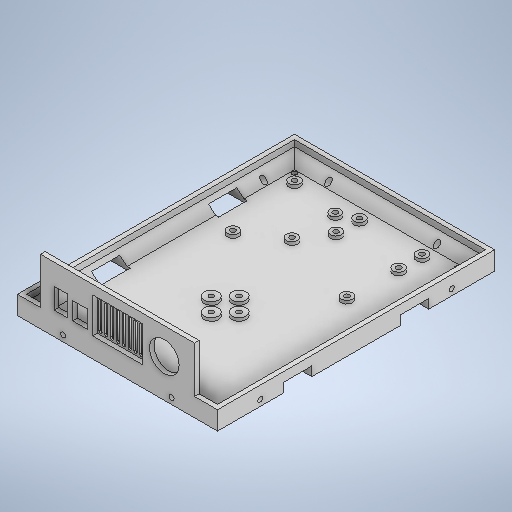
# Autodesk Inventor part: base_v2
Saved by Autodesk Inventor 2025.1 (Build 291241000, 241)
## iProperties
Created: 2024-08-06
Part Number: base_v2
Material: Genérico
Document SubType Name: Modeling
Designer: andre
Density: 1 g/cm^3
Appearance: Valor por defecto
Author: andre
Autodesk Inventor part; units mm, degrees
ref_plane "YZ Plane" through (0, 0, 0) normal (1, 0, 0) x (0, 1, 0)
ref_plane "XZ Plane" through (0, 0, 0) normal (0, 1, 0) x (-1, 0, 0)
ref_plane "XY Plane" through (0, 0, 0) normal (0, 0, 1) x (1, 0, 0)
sketch "base" plane through (0, 0, 0) normal (0, 1, 0) x (-1, 0, 0)
  line L0 (0, 0) -> (130, 0)
  line L1 (130, 0) -> (130, -180)
  line L2 (130, -180) -> (0, -180)
  line L3 (0, -180) -> (0, 0)
  dimension "d53" = 130
  dimension "d54" = 180
  constraints: 8 end point, 2 parallel, 1 horizontal, 1 perpendicular
  measures "d53" distance of L1.end L2.end
  measures "d54" distance of L0.end L1.end
extrude "Extrusión6" add sketch "base" along normal blind 2
sketch "Boceto10" plane through (0, 2, 0) normal (0, 1, 0) x (1, 0, 0)
  line L0 (-130, 180) -> (-130, 0) projected
  line L1 (0, 180) -> (-130, 180) projected
  line L2 (-130, 0) -> (0, 0)
  line L3 (0, 0) -> (0, 180)
  line L4 (0, 180) -> (-130, 180)
  line L5 (-130, 180) -> (-130, 0)
  line L6 (-3, 3) -> (-127, 3)
  line L7 (-127, 3) -> (-127, 177)
  line L8 (-127, 177) -> (-3, 177)
  line L9 (-3, 177) -> (-3, 3)
  dimension "d57" = 3
  constraints: 16 end point, 4 parallel, 2 perpendicular, 1 horizontal, 3 other
  measures "d57" distance between parallel lines of L2 L6
extrude "Extrusión7" add sketch "Boceto10" along normal blind 10
sketch "Boceto17" plane through (0, 12, 0) normal (0, 1, 0) x (1, 0, 0)
  line L0 (-3, 177) -> (-3, 3) projected
  line L1 (0, 0) -> (0, 180) construction
  line L2 (-3, 3) -> (-127, 3) construction
  line L3 (0, 0) -> (-15, 0) construction
  line L4 (-15, 0) -> (-15, 3) construction
  line L5 (-15, 3) -> (0, 3) construction
  line L6 (0, 3) -> (0, 0) construction
  line L7 (-130, 180) -> (-130, 0) construction
  line L8 (-130, 0) -> (-115, 0) construction
  line L9 (-115, 0) -> (-115, 3) construction
  line L10 (-115, 3) -> (-130, 3) construction
  line L11 (-130, 3) -> (-130, 0) construction
  line L12 (-15, 0) -> (-115, 0)
  line L13 (-115, 0) -> (-115, 3)
  line L14 (-115, 3) -> (-15, 3)
  line L15 (-15, 3) -> (-15, 0)
  dimension "d176" = 15
  dimension "d177" = 15
  constraints: 24 end point, 6 parallel, 3 horizontal, 3 perpendicular, 2 point on line
  measures "d176" distance of L4.end L5.end
  measures "d177" distance of L10.end L9.end
extrude "Extrusión13" add sketch "Boceto17" along normal blind 30
sketch "Boceto16" plane through (0, 2, 0) normal (0, 1, 0) x (1, 0, 0)
  line L0 (-3, 177) -> (-127, 177) projected
  line L1 (-3, 3) -> (-3, 177) projected
  line L2 (-127, 177) -> (-3, 177)
  line L3 (-3, 177) -> (-3, 3)
  line L4 (-3, 3) -> (-127, 3)
  line L5 (-127, 3) -> (-127, 177)
  line L6 (-120, 170) -> (-10, 170)
  line L7 (-10, 170) -> (-10, 10)
  line L8 (-10, 10) -> (-120, 10)
  line L9 (-120, 10) -> (-120, 170)
  point P0 (0, 0)
  dimension "d170" = 7
  constraints: 16 end point, 4 parallel, 2 perpendicular, 1 horizontal, 3 other
  measures "d170" distance between parallel lines of L5 L9
extrude "Extrusión12" add sketch "Boceto16" along normal blind 6
sketch "Boceto15" plane through (0, 0, 0) normal (0, -1, 0) x (1, 0, 0)
  line L0 (-130, 0) -> (0, 0) projected
  line L1 (-130, -180) -> (-130, 0) projected
  line L2 (0, 0) -> (-130, 0)
  line L3 (-130, 0) -> (-130, -180)
  line L4 (-130, -180) -> (0, -180)
  line L5 (0, -180) -> (0, 0)
  line L6 (0, -180) -> (-1.1, -180) construction
  line L7 (0, -157.5704) -> (0, -180) construction
  line L8 (0, -180) -> (-12, -180) construction
  line L9 (-12, -180) -> (-12, -168) construction
  line L10 (-12, -168) -> (0, -168) construction
  line L11 (0, -168) -> (0, -180) construction
  line L12 (0, 0) -> (-12, 0) construction
  line L13 (-12, 0) -> (-12, -12) construction
  line L14 (-12, -12) -> (0, -12) construction
  line L15 (0, -12) -> (0, 0) construction
  line L16 (-130, 0) -> (-118, 0) construction
  line L17 (-118, 0) -> (-118, -12) construction
  line L18 (-118, -12) -> (-130, -12) construction
  line L19 (-130, -12) -> (-130, 0) construction
  line L20 (-130, -180) -> (-118, -180) construction
  line L21 (-118, -180) -> (-118, -168) construction
  line L22 (-118, -168) -> (-130, -168) construction
  line L23 (-130, -168) -> (-130, -180) construction
  circle A0 centre (-12, -168) radius 1.625
  circle A1 centre (-118, -168) radius 1.625
  circle A2 centre (-12, -12) radius 1.625
  circle A3 centre (-118, -12) radius 1.625
  dimension "d155" = 12
  dimension "d156" = 12
  dimension "d157" = 12
  dimension "d158" = 12
  dimension "d159" = 12
  dimension "d160" = 12
  dimension "d161" = 12
  dimension "d162" = 12
  dimension "d163" = 3.25
  dimension "d164" = 3.25
  dimension "d165" = 3.25
  dimension "d166" = 3.25
  constraints: 44 end point, 10 parallel, 6 horizontal, 5 perpendicular, 4 centre point, 4 coincident
  measures "d155" distance of L9.end L10.end
  measures "d156" distance of L8.end L9.end
  measures "d157" distance of L14.end L13.end
  measures "d158" distance of L13.end L12.end
  measures "d159" distance of L17.end L18.end
  measures "d160" distance of L16.end L17.end
  measures "d161" distance of L22.end L21.end
  measures "d162" distance of L21.end L20.end
  measures "d163" diameter of A0
  measures "d164" diameter of A1
  measures "d165" diameter of A2
  measures "d166" diameter of A3
extrude "Extrusión11" cut sketch "Boceto15" against normal blind 30 contours A0 | A1 | A2 | A3
sketch "Boceto11" plane through (0, 2, 0) normal (0, 1, 0) x (1, 0, 0)
  line L0 (-127, 3) -> (-127, 177) projected
  line L1 (-3, 177) -> (-3, 3) projected
  line L2 (-127, 3) -> (-3, 3)
  line L3 (-3, 3) -> (-3, 177)
  line L4 (-3, 177) -> (-127, 177)
  line L5 (-127, 177) -> (-127, 3)
  line L6 (-130, 0) -> (0, 0) projected
  line L7 (-130, 0) -> (0, 0)
  line L8 (0, 0) -> (0, 180.7986)
  line L9 (0, 180.7986) -> (-130, 180.7986)
  line L10 (-130, 180.7986) -> (-130, 0)
  line L11 (-9, 9) -> (-121, 9) construction
  line L12 (-121, 9) -> (-121, 171) construction
  line L13 (-121, 171) -> (-9, 171) construction
  line L14 (-9, 171) -> (-9, 9) construction
  line L15 (-121, 171) -> (-9, 171) construction
  line L16 (-9, 171) -> (-9, 108) construction
  line L17 (-9, 108) -> (-121, 108) construction
  line L18 (-121, 108) -> (-121, 171) construction
  line L19 (-118, 111) -> (-16, 111) construction
  line L20 (-16, 111) -> (-16, 165) construction
  line L21 (-16, 165) -> (-118, 165) construction
  line L22 (-118, 165) -> (-118, 111) construction
  line L23 (-121, 108) -> (-117.6431, 108) construction
  line L24 (-16, 165) -> (-30, 165) construction
  line L25 (-30, 165) -> (-30, 162) construction
  line L26 (-30, 162) -> (-16, 162) construction
  line L27 (-16, 162) -> (-16, 165) construction
  line L28 (-30, 162) -> (-30, 114) construction
  line L29 (-30, 162) -> (18, 162) construction
  line L30 (-30, 162) -> (-112, 162) construction
  line L31 (-30, 162) -> (52, 162) construction
  line L32 (-30, 114) -> (-104, 114) construction
  line L33 (-30, 114) -> (44, 114) construction
  circle A0 centre (-104, 114) radius 1.625 construction
  circle A1 centre (-112, 162) radius 1.625 construction
  circle A2 centre (-30, 114) radius 1.625 construction
  line L34 (-30, 114) -> (-80.8, 114) construction
  line L35 (-80.8, 114) -> (-80.8, 129.2) construction
  line L36 (-80.8, 129.2) -> (-30, 129.2) construction
  line L37 (-30, 129.2) -> (-30, 114) construction
  circle A3 centre (-80.8, 129.2) radius 1.625 construction
  line L38 (-30, 162) -> (-80.8, 162) construction
  line L39 (-80.8, 162) -> (-80.8, 157.3) construction
  line L40 (-80.8, 157.3) -> (-30, 157.3) construction
  line L41 (-30, 157.3) -> (-30, 162) construction
  circle A4 centre (-80.8, 157.3) radius 1.5 construction
  line L42 (-30, 162) -> (-29.1, 162) construction
  circle A5 centre (-29.1, 162) radius 1.625 construction
  line L43 (-65, 9) -> (-65, 70) construction
  line L44 (-65, 9) -> (-4, 9) construction
  line L45 (-29.1, 162) -> (-69.74, 162) construction
  line L46 (-69.74, 162) -> (-69.74, 146.76) construction
  line L47 (-69.74, 146.76) -> (-29.1, 146.76) construction
  line L48 (-29.1, 146.76) -> (-29.1, 162) construction
  circle A6 centre (-69.74, 146.76) radius 1.625 construction
  circle A7 centre (-69.74, 162) radius 1.625 construction
  circle A8 centre (-29.1, 146.76) radius 1.625 construction
  circle A9 centre (-65, 70) radius 9 construction
  circle A10 centre (-65, 70) radius 51 construction
  circle A11 centre (-65, 70) radius 45 construction
  circle A12 centre (-65, 61) radius 1.625 construction
  line L49 (-65, 61) -> (-65, 79) construction
  circle A13 centre (-65, 79) radius 1.625 construction
  circle A14 centre (-56, 70) radius 1.625 construction
  circle A15 centre (-74, 70) radius 1.625 construction
  circle A16 centre (-65, 61) radius 4.625
  circle A17 centre (-74, 70) radius 4.625
  circle A18 centre (-65, 79) radius 4.625
  circle A19 centre (-56, 70) radius 4.625
  circle A20 centre (-30, 114) radius 3.625
  circle A21 centre (-29.1, 146.76) radius 3.625
  circle A22 centre (-104, 114) radius 3.625
  circle A23 centre (-80.8, 129.2) radius 3.625
  circle A24 centre (-112, 162) radius 3.625
  circle A25 centre (-80.8, 157.3) radius 3.5
  circle A26 centre (-69.74, 146.76) radius 3.625
  circle A27 centre (-69.74, 162) radius 3.625
  circle A28 centre (-29.1, 162) radius 3.625
  point P0 (-118, 111)
  point P1 (-27.9651, 111)
  point P2 (-32.0349, 111)
  point P3 (-31.1349, 165)
  point P4 (-27.0651, 165)
  point P5 (-71.7749, 165)
  point P6 (-67.7051, 165)
  point P7 (-114.0349, 165)
  point P8 (-109.9651, 165)
  dimension "d60" = 6
  dimension "d64" = 102
  dimension "d65" = 54
  dimension "d71" = 3
  dimension "d73" = 3
  dimension "d74" = 14
  dimension "d75" = 3
  dimension "d76" = 48
  dimension "d78" = 82
  dimension "d80" = 74
  dimension "d86" = 50.8
  dimension "d87" = 15.2
  dimension "d88" = 3.25
  dimension "d89" = 50.8
  dimension "d90" = 4.7
  dimension "d91" = 3
  dimension "d92" = 0.9
  dimension "d96" = 61
  dimension "d97" = 40.64
  dimension "d98" = 15.24
  dimension "d99" = 3.25
  dimension "d100" = 3.25
  dimension "d101" = 3.25
  dimension "d102" = 18
  dimension "d103" = 102
  dimension "d104" = 6
  dimension "d105" = 3.25
  dimension "d106" = 3.25
  dimension "d107" = 3.25
  dimension "d108" = 3.25
  dimension "d109" = 3
  dimension "d110" = 3
  dimension "d111" = 3
  dimension "d112" = 3
  dimension "d113" = 2
  dimension "d114" = 2
  dimension "d115" = 2
  dimension "d116" = 2
  dimension "d117" = 2
  dimension "d118" = 2
  dimension "d119" = 2
  dimension "d120" = 2
  dimension "d121" = 2
  dimension "d380" = 3.25
  dimension "d381" = 3.25
  dimension "d382" = 3.25
  dimension "d383" = 3.25
  constraints: 94 end point, 29 centre point, 23 coincident, 18 parallel, 15 horizontal, 10 perpendicular, 4 equal length, 4 point on circle, 3 point on line, 1 midpoint, 1 vertical, 3 other
  measures "d60" distance between parallel lines of L2 L11
  measures "d64" distance of L21.end L20.end
  measures "d65" distance of L20.end L19.end
  measures "d71" distance from line of L18 point (-118, 111)
  measures "d73" distance from line of L23 point (-118, 111)
  measures "d74" distance of L26.end L25.end
  measures "d75" distance of L25.end L24.end
  measures "d76" distance of L28.start L28.end
  measures "d78" distance of L28.start L30.end
  measures "d80" distance of L32.start L32.end
  measures "d86" distance of L35.end L36.end
  measures "d87" distance of L34.end L35.end
  measures "d88" diameter of A3
  measures "d89" distance of L40.end L39.end
  measures "d90" distance of L39.end L38.end
  measures "d91" diameter of A4
  measures "d92" distance of L38.start L42.end
  measures "d96" distance of point (-65, 70) L43.start
  measures "d97" distance of L47.end L46.end
  measures "d98" distance of L46.end L45.end
  measures "d99" diameter of A6
  measures "d100" diameter of A7
  measures "d101" diameter of A8
  measures "d102" diameter of A9
  measures "d103" diameter of A10
  measures "d104" radial gap between concentric circles of A10 A11
  measures "d105" diameter of A12
  measures "d106" diameter of A13
  measures "d107" diameter of A14
  measures "d108" diameter of A15
  measures "d109" radial gap between concentric circles of A12 A16
  measures "d110" radial gap between concentric circles of A15 A17
  measures "d111" radial gap between concentric circles of A13 A18
  measures "d112" radial gap between concentric circles of A14 A19
  measures "d113" radial gap between concentric circles of A2 A20
  measures "d114" radial gap between concentric circles of A8 A21
  measures "d115" radial gap between concentric circles of A0 A22
  measures "d116" radial gap between concentric circles of A3 A23
  measures "d117" radial gap between concentric circles of A1 A24
  measures "d118" radial gap between concentric circles of A4 A25
  measures "d119" radial gap between concentric circles of A6 A26
  measures "d120" radial gap between concentric circles of A7 A27
  measures "d121" radial gap between concentric circles of A5 A28
  measures "d380" diameter of A5
  measures "d381" diameter of A1
  measures "d382" diameter of A0
  measures "d383" diameter of A2
extrude "Extrusión8" add sketch "Boceto11" along normal blind 2 contours A16 | A17 | A18 | A19 | A20 | A21 | A22 | A23 | A24 | A25 | A26 | A27 | A28
chamfer "Chaflán1" distance 7 distance2 6 4 edges at (-120, 8, -90) (-65, 8, -170) (-10, 8, -90) (-65, 8, -10) measured on face at (-124.6667, 8, -116.6667)
sketch "Boceto20" plane through (-130, 0, -180) normal (-1, 0, 0) x (0, 0, 1)
  line L0 (180, 0) -> (0, 0) projected
  line L1 (177, 12) -> (3, 12) projected
  line L2 (3, 8) -> (177, 8) projected
  line L3 (3, 8) -> (177, 8)
  line L4 (90, 8) -> (90, 0) construction
  line L5 (180, 0) -> (180, 12) construction
  circle A0 centre (27.8, 4) radius 1.625
  circle A1 centre (152.2, 4) radius 1.625
  line L6 (180, 0) -> (152.2, 0) construction
  line L7 (152.2, 0) -> (152.2, 4) construction
  line L8 (152.2, 4) -> (180, 4) construction
  line L9 (180, 4) -> (180, 0) construction
  point P0 (90, 4)
  point P1 (90, 12)
  dimension "d237" = 3.25
  dimension "d238" = 3.25
  dimension "d307" = 62.2
  dimension "d308" = 62.2
  dimension "d405" = 4
  dimension "d406" = 4
  constraints: 12 end point, 4 midpoint, 2 centre point, 2 horizontal, 2 parallel, 2 perpendicular
  measures "d237" diameter of A0
  measures "d238" diameter of A1
  measures "d307" distance of point (90, 4) A0.centre
  measures "d308" distance from line of L7.end L4
  measures "d405" distance from line of L0 L7.end
  measures "d406" distance from line of L0 A0.centre
extrude "Extrusión16" cut sketch "Boceto20" against normal blind 140
sketch "Boceto18" plane through (-130, 0, 0) normal (0, 0, 1) x (1, 0, 0)
  line L0 (0, 42) -> (0, 0) construction
  line L1 (0, 0) -> (35, 0) construction
  line L2 (36, 15) -> (45.4, 15)
  line L3 (45.4, 15) -> (45.4, 26.4)
  line L4 (45.4, 26.4) -> (36, 26.4)
  line L5 (36, 26.4) -> (36, 15)
  line L6 (130, 0) -> (95.45, 0) construction
  line L7 (95.45, 0) -> (95.45, 24.65) construction
  line L8 (95.45, 24.65) -> (130, 24.65) construction
  line L9 (130, 24.65) -> (130, 0) construction
  circle A0 centre (95.45, 24.65) radius 9.65
  line L10 (0, 0) -> (130, 0) construction
  line L11 (130, 0) -> (130, 60) construction
  line L12 (130, 60) -> (0, 60) construction
  line L13 (0, 60) -> (0, 0) construction
  line L14 (23, 0) -> (1, 0) construction
  line L15 (24, 15) -> (32.4, 15)
  line L16 (32.4, 15) -> (32.4, 28.4)
  line L17 (32.4, 28.4) -> (24, 28.4)
  line L18 (24, 28.4) -> (24, 15)
  line L19 (20, 37) -> (110, 37)
  line L20 (110, 12) -> (20, 12)
  line L21 (20, 37) -> (20, 12)
  line L22 (110, 37) -> (110, 12)
  line L23 (42.5275, 15) -> (41.0275, 15)
  line L24 (20, 15) -> (110, 15) construction
  line L25 (85.8, 24.65) -> (85.8, 15) construction
  line L26 (50, 15) -> (79.4, 15) construction
  line L27 (50.9, 33.1) -> (50.9, 16)
  line L28 (52.9, 16) -> (52.9, 33.1)
  arc A1 (50.9, 16) -> (52.9, 16) centre (51.9, 16) ccw
  arc A2 (52.9, 33.1) -> (50.9, 33.1) centre (51.9, 33.1) ccw
  line L29 (54.7, 33.1) -> (54.7, 16)
  line L30 (56.7, 16) -> (56.7, 33.1)
  arc A3 (54.7, 16) -> (56.7, 16) centre (55.7, 16) ccw
  line L31 (58.5, 33.1) -> (58.5, 16)
  line L32 (60.5, 16) -> (60.5, 33.1)
  arc A4 (58.5, 16) -> (60.5, 16) centre (59.5, 16) ccw
  arc A5 (60.5, 33.1) -> (58.5, 33.1) centre (59.5, 33.1) ccw
  arc A6 (62.3, 16) -> (64.3, 16) centre (63.3, 16) ccw
  line L33 (64.3, 16) -> (64.3, 33.1)
  line L34 (62.3, 33.1) -> (62.3, 16)
  line L35 (66.1, 33.1) -> (66.1, 16)
  line L36 (68.1, 16) -> (68.1, 33.1)
  arc A7 (66.1, 16) -> (68.1, 16) centre (67.1, 16) ccw
  arc A8 (68.1, 33.1) -> (66.1, 33.1) centre (67.1, 33.1) ccw
  arc A9 (69.9, 16) -> (71.9, 16) centre (70.9, 16) ccw
  line L37 (71.9, 16) -> (71.9, 33.1)
  line L38 (69.9, 33.1) -> (69.9, 16)
  line L39 (73.7, 33.1) -> (73.7, 16)
  line L40 (75.7, 16) -> (75.7, 33.1)
  arc A10 (73.7, 16) -> (75.7, 16) centre (74.7, 16) ccw
  arc A11 (75.7, 33.1) -> (73.7, 33.1) centre (74.7, 33.1) ccw
  arc A12 (77.5, 16) -> (79.5, 16) centre (78.5, 16) ccw
  line L41 (79.5, 16) -> (79.5, 33.1)
  line L42 (77.5, 33.1) -> (77.5, 16)
  arc A13 (56.7, 33.1) -> (54.7, 33.1) centre (55.7, 33.1) ccw
  arc A14 (64.3, 33.1) -> (62.3, 33.1) centre (63.3, 33.1) ccw
  arc A15 (71.9, 33.1) -> (69.9, 33.1) centre (70.9, 33.1) ccw
  arc A16 (79.5, 33.1) -> (77.5, 33.1) centre (78.5, 33.1) ccw
  point P0 (95.45, 15)
  point P1 (105.1, 24.65)
  point P2 (95.45, 15)
  dimension "d182" = 9.4
  dimension "d186" = 34.55
  dimension "d188" = 19.3
  dimension "d189" = 60
  dimension "d190" = 15
  dimension "d191" = 8.4
  dimension "d192" = 13.4
  dimension "d193" = 23
  dimension "d195" = 12
  dimension "d196" = 20
  dimension "d198" = 20
  dimension "d201" = 15
  dimension "d202" = 24
  dimension "d203" = 15
  dimension "d204" = 36
  dimension "d205" = 1.5
  dimension "d207" = 50
  dimension "d250" = 25
  dimension "d407" = 11.4
  dimension "d408" = 2
  dimension "d409" = 2
  dimension "d410" = 2
  dimension "d411" = 2
  dimension "d412" = 2
  dimension "d413" = 2
  dimension "d414" = 2
  dimension "d415" = 2
  dimension "d424" = 5.5
  dimension "d425" = 1.8
  dimension "d426" = 1.8
  dimension "d427" = 1.8
  dimension "d428" = 1.8
  dimension "d429" = 1.8
  dimension "d430" = 1.8
  dimension "d431" = 1.8
  constraints: 90 end point, 35 point on circle, 25 tangent, 17 centre point, 17 parallel, 7 perpendicular, 7 point on line, 6 horizontal, 3 coincident, 1 vertical
  measures "d182" distance of L4.end L3.end
  measures "d186" distance of L7.end L8.end
  measures "d188" diameter of A0
  measures "d189" distance of L11.end L10.end
  measures "d190" distance of L6.end point (95.45, 15)
  measures "d191" distance of L17.end L16.end
  measures "d192" distance of L16.end L15.end
  measures "d193" distance between parallel lines of L12 L19
  measures "d195" distance between parallel lines of L10 L20
  measures "d196" distance between parallel lines of L21 L0
  measures "d198" distance between parallel lines of L9 L22
  measures "d201" distance between parallel lines of L1 L15
  measures "d202" distance between parallel lines of L0 L18
  measures "d203" distance between parallel lines of L10 L2
  measures "d204" distance between parallel lines of L0 L5
  measures "d205" distance of L23.start L23.end
  measures "d207" distance from line of L0 L26.start
  measures "d250" distance between parallel lines of L20 L19
  measures "d407" distance between parallel lines of L4 L2
  measures "d408" distance between parallel lines of L28 L27
  measures "d409" distance between parallel lines of L30 L29
  measures "d410" distance between parallel lines of L32 L31
  measures "d411" distance between parallel lines of L33 L34
  measures "d412" distance between parallel lines of L36 L35
  measures "d413" distance between parallel lines of L37 L38
  measures "d414" distance between parallel lines of L40 L39
  measures "d415" distance between parallel lines of L41 L42
  measures "d424" distance between parallel lines of L3 L27
  measures "d425" distance between parallel lines of L29 L28
  measures "d426" distance between parallel lines of L30 L31
  measures "d427" distance between parallel lines of L34 L32
  measures "d428" distance between parallel lines of L33 L35
  measures "d429" distance between parallel lines of L38 L36
  measures "d430" distance between parallel lines of L37 L39
  measures "d431" distance between parallel lines of L40 L42
extrude "Extrusión14" cut sketch "Boceto18" against normal blind 10 contours L5 L4 L3 L2 | A0 | L18 L17 L16 L15 | A2 L28 A1 L27 | A13 L30 A3 L29 | A5 L32 A4 L31 | L34 A14 L33 A6 | A8 L36 A7 L35 | L38 A15 L37 A9 | A11 L40 A10 L39 | L42 A16 L41 A12
sketch "Boceto12" plane through (-30, 4, -114) normal (0, 1, 0) x (1, 0, 0)
  circle A0 centre (0, 0) radius 3.625
  circle A1 centre (-35, -35) radius 4.625 projected
  circle A2 centre (-35, -35) radius 4.5
  circle A3 centre (-26, -44) radius 4.625 projected
  circle A4 centre (-26, -44) radius 4.5
  circle A5 centre (-35, -53) radius 4.625 projected
  circle A6 centre (-35, -53) radius 4.5
  circle A7 centre (-44, -44) radius 4.625 projected
  circle A8 centre (-44, -44) radius 4.5
  circle A9 centre (0.9, 32.76) radius 3.625 projected
  circle A10 centre (0.9, 32.76) radius 3.5
  circle A11 centre (0.9, 48) radius 3.625 projected
  circle A12 centre (0.9, 48) radius 3.5
  circle A13 centre (-39.74, 32.76) radius 3.625 projected
  circle A14 centre (-39.74, 32.76) radius 3.625
  circle A15 centre (-39.74, 48) radius 3.625 projected
  circle A16 centre (-39.74, 48) radius 3.625
  circle A17 centre (-50.8, 43.3) radius 3.5 projected
  circle A18 centre (-50.8, 43.3) radius 3.5
  circle A19 centre (-50.8, 15.2) radius 3.625 projected
  circle A20 centre (-50.8, 15.2) radius 3.5
  circle A21 centre (-74, 0) radius 3.625 projected
  circle A22 centre (-74, 0) radius 3.5
  circle A23 centre (-82, 48) radius 3.625 projected
  circle A24 centre (-82, 48) radius 3.5
  circle A25 centre (-82, 48) radius 1.625
  circle A26 centre (-74, 0) radius 1.625
  circle A27 centre (-50.8, 15.2) radius 1.625
  circle A28 centre (-39.74, 32.76) radius 1.625
  circle A29 centre (-39.74, 48) radius 1.625
  circle A30 centre (-50.8, 43.3) radius 1.625
  circle A31 centre (-44, -44) radius 1.625
  circle A32 centre (-35, -53) radius 1.625
  circle A33 centre (-35, -35) radius 1.625
  circle A34 centre (-26, -44) radius 1.625
  circle A35 centre (0, 0) radius 1.625
  circle A36 centre (0.9, 32.76) radius 1.625
  circle A37 centre (0.9, 48) radius 1.625
  point P0 (30, -114)
  dimension "d124" = 2
  dimension "d125" = 2
  dimension "d126" = 2
  dimension "d127" = 2
  dimension "d128" = 2
  dimension "d130" = 3
  dimension "d131" = 3
  dimension "d132" = 3
  dimension "d133" = 3
  dimension "d134" = 2
  dimension "d135" = 2
  dimension "d136" = 2
  dimension "d385" = 3.25
  dimension "d386" = 3.25
  dimension "d387" = 3.25
  dimension "d395" = 3.25
  constraints: 26 centre point, 12 coincident
  measures "d124" radial gap between concentric circles of A23 A25
  measures "d125" radial gap between concentric circles of A21 A26
  measures "d126" radial gap between concentric circles of A19 A27
  measures "d127" radial gap between concentric circles of A14 A28
  measures "d128" radial gap between concentric circles of A16 A29
  measures "d130" radial gap between concentric circles of A7 A31
  measures "d131" radial gap between concentric circles of A5 A32
  measures "d132" radial gap between concentric circles of A1 A33
  measures "d133" radial gap between concentric circles of A3 A34
  measures "d134" radial gap between concentric circles of A0 A35
  measures "d135" radial gap between concentric circles of A9 A36
  measures "d136" radial gap between concentric circles of A11 A37
  measures "d385" diameter of A28
  measures "d386" diameter of A29
  measures "d387" diameter of A35
  measures "d395" diameter of A30
extrude "Extrusión9" cut sketch "Boceto12" along normal mid plane 30 contours A25 | A26 | A27 | A28 | A29 | A30 | A31 | A32 | A33 | A34 | A35 | A36 | A37
sketch "Boceto13" plane through (0, 0, 0) normal (0, -1, 0) x (1, 0, 0)
  circle A0 centre (-112, -162) radius 1.625 projected
  circle A1 centre (-112, -162) radius 1.625
  circle A2 centre (-80.8, -157.3) radius 1.625 projected
  circle A3 centre (-80.8, -157.3) radius 1.625
  circle A4 centre (-69.74, -162) radius 1.625 projected
  circle A5 centre (-69.74, -162) radius 1.625
  circle A6 centre (-69.74, -146.76) radius 1.625 projected
  circle A7 centre (-69.74, -146.76) radius 1.625
  circle A8 centre (-80.8, -129.2) radius 1.625 projected
  circle A9 centre (-80.8, -129.2) radius 1.625
  circle A10 centre (-104, -114) radius 1.625 projected
  circle A11 centre (-104, -114) radius 1.625
  circle A12 centre (-74, -70) radius 1.625 projected
  circle A13 centre (-74, -70) radius 1.625
  circle A14 centre (-65, -79) radius 1.625 projected
  circle A15 centre (-65, -79) radius 1.625
  circle A16 centre (-56, -70) radius 1.625 projected
  circle A17 centre (-56, -70) radius 1.625
  circle A18 centre (-65, -61) radius 1.625 projected
  circle A19 centre (-65, -61) radius 1.625
  circle A20 centre (-112, -162) radius 3.325
  circle A21 centre (-80.8, -157.3) radius 3.325
  circle A22 centre (-69.74, -162) radius 3.325
  circle A23 centre (-69.74, -146.76) radius 3.325
  circle A24 centre (-80.8, -129.2) radius 3.325
  circle A25 centre (-104, -114) radius 3.325
  circle A26 centre (-74, -70) radius 3.325
  circle A27 centre (-65, -79) radius 3.325
  circle A28 centre (-65, -61) radius 3.325
  circle A29 centre (-56, -70) radius 3.325
  circle A30 centre (-29.1, -162) radius 3.625 projected
  circle A31 centre (-29.1, -162) radius 1.625
  circle A32 centre (-29.1, -146.76) radius 1.625 projected
  circle A33 centre (-29.1, -146.76) radius 1.625
  circle A34 centre (-30, -114) radius 1.625 projected
  circle A35 centre (-30, -114) radius 1.625
  circle A36 centre (-29.1, -162) radius 3.325
  circle A37 centre (-29.1, -146.76) radius 3.325
  circle A38 centre (-30, -114) radius 3.325
  point P0 (0, 0)
  dimension "d139" = 1.7
  dimension "d140" = 1.7
  dimension "d141" = 1.7
  dimension "d142" = 1.7
  dimension "d143" = 1.7
  dimension "d144" = 1.7
  dimension "d145" = 1.7
  dimension "d146" = 1.7
  dimension "d147" = 1.7
  dimension "d148" = 1.7
  dimension "d149" = 1.7
  dimension "d150" = 1.7
  dimension "d151" = 1.7
  dimension "d388" = 3.25
  dimension "d389" = 3.25
  dimension "d390" = 3.25
  dimension "d391" = 3.25
  dimension "d393" = 3.25
  dimension "d396" = 3.25
  dimension "d397" = 3.25
  dimension "d398" = 3.25
  dimension "d399" = 3.25
  dimension "d400" = 3.25
  dimension "d401" = 3.25
  dimension "d402" = 3.25
  dimension "d403" = 3.25
  dimension "d404" = 3.25
  constraints: 26 centre point, 13 coincident
  measures "d139" radial gap between concentric circles of A0 A20
  measures "d140" radial gap between concentric circles of A2 A21
  measures "d141" radial gap between concentric circles of A4 A22
  measures "d142" radial gap between concentric circles of A6 A23
  measures "d143" radial gap between concentric circles of A9 A24
  measures "d144" radial gap between concentric circles of A11 A25
  measures "d145" radial gap between concentric circles of A12 A26
  measures "d146" radial gap between concentric circles of A14 A27
  measures "d147" radial gap between concentric circles of A18 A28
  measures "d148" radial gap between concentric circles of A16 A29
  measures "d149" radial gap between concentric circles of A31 A36
  measures "d150" radial gap between concentric circles of A32 A37
  measures "d151" radial gap between concentric circles of A34 A38
  measures "d388" diameter of A31
  measures "d389" diameter of A33
  measures "d390" diameter of A5
  measures "d391" diameter of A7
  measures "d393" diameter of A6
  measures "d396" diameter of A1
  measures "d397" diameter of A3
  measures "d398" diameter of A9
  measures "d399" diameter of A35
  measures "d400" diameter of A11
  measures "d401" diameter of A15
  measures "d402" diameter of A13
  measures "d403" diameter of A19
  measures "d404" diameter of A17
extrude "Extrusión10" cut sketch "Boceto13" against normal blind 1 contours A20 | A21 | A22 | A23 | A24 | A25 | A26 | A27 | A28 | A29 | A36 | A37 | A38
sketch "Boceto19" plane through (-130, 0, 0) normal (0, 0, 1) x (1, 0, 0)
  arc A0 (52.9, 33.1) -> (50.9, 33.1) centre (51.9, 33.1) ccw construction
  arc A1 (77.5, 16) -> (79.5, 16) centre (78.5, 16) ccw construction
  line L0 (51.9, 33.1) -> (78.5, 33.1) construction
  line L1 (78.5, 33.1) -> (78.5, 16) construction
  line L2 (78.5, 16) -> (51.9, 16) construction
  line L3 (51.9, 16) -> (51.9, 33.1) construction
  line L4 (80.5, 14) -> (80.5, 35.1)
  line L5 (80.5, 35.1) -> (49.9, 35.1)
  line L6 (49.9, 35.1) -> (49.9, 14)
  line L7 (49.9, 14) -> (80.5, 14)
  point P0 (130, 0)
  dimension "d226" = 2
  constraints: 16 end point, 4 parallel, 2 perpendicular, 1 horizontal, 3 other
  measures "d226" distance between parallel lines of L1 L4
extrude "Extrusión15" cut sketch "Boceto19" against normal blind 2
sketch "Boceto21" plane through (-130, 0, 0) normal (0, 0, 1) x (1, 0, 0)
  line L0 (127, 8) -> (3, 8) construction
  line L1 (3, 8) -> (127, 8)
  line L2 (130, 0) -> (0, 0) projected
  line L3 (65, 8) -> (65, 0) construction
  line L4 (130, 0) -> (130, 12) construction
  circle A0 centre (29.8, 4) radius 1.625
  circle A1 centre (100.2, 4) radius 1.625
  point P0 (65, 4)
  dimension "d239" = 3.25
  dimension "d240" = 3.25
  dimension "d248" = 4
  dimension "d323" = 35.2
  dimension "d324" = 35.2
  constraints: 4 end point, 3 midpoint, 2 centre point, 2 coincident, 1 collinear, 1 perpendicular
  measures "d239" diameter of A0
  measures "d240" diameter of A1
  measures "d248" distance from line of L2 point (29.8, 4)
  measures "d323" distance of point (65, 4) A0.centre
  measures "d324" distance of A1.centre point (65, 4)
extrude "Extrusión17" cut sketch "Boceto21" against normal blind 20
sketch "Boceto22" plane through (0, 0, -180) normal (0, 0, -1) x (-1, 0, 0)
  line L0 (3, 8) -> (127, 8) construction
  line L1 (3, 8) -> (127, 8) construction
  line L2 (0, 0) -> (130, 0) construction
  line L3 (65, 8) -> (65, 0) construction
  line L4 (120, 2) -> (10, 2) construction
  circle A0 centre (29.8, 4) radius 1.625
  circle A1 centre (100.2, 4) radius 1.625
  line L5 (0, 0) -> (29.8, 0) construction
  line L6 (29.8, 0) -> (29.8, 4) construction
  line L7 (0, 4) -> (0, 0) construction
  line L8 (100.2, 4) -> (130, 4) construction
  line L9 (130, 4) -> (130, 0) construction
  line L10 (130, 0) -> (100.2, 0) construction
  line L11 (100.2, 0) -> (100.2, 4) construction
  point P0 (65, 4)
  dimension "d243" = 3.25
  dimension "d244" = 3.25
  dimension "d247" = 4
  dimension "d327" = 35.2
  dimension "d328" = 35.2
  constraints: 18 end point, 3 horizontal, 3 midpoint, 3 parallel, 3 perpendicular, 2 centre point, 2 coincident
  measures "d243" diameter of A0
  measures "d244" diameter of A1
  measures "d247" distance from line of L2 L6.end
  measures "d327" distance of point (65, 4) L6.end
  measures "d328" distance of point (65, 4) L8.start
extrude "Extrusión18" cut sketch "Boceto22" against normal blind 12
chamfer "Chaflán2" distance 1 distance2 2 4 edges at (-80.1, 24.55, 0) (-64.8, 35.1, 0) (-49.5, 24.55, 0) (-64.8, 14, 0) measured on face at (-70.0333, 6.615, 0)
sketch "Boceto23" plane through (0, 0, 0) normal (1, 0, 0) x (0, 0, -1)
  line L0 (0, 0) -> (180, 0) projected
  line L1 (3, 12) -> (177, 12) projected
  line L2 (90, 0) -> (90, 12) construction
  line L3 (90, 0) -> (74.0707, 0)
  line L4 (52, 0) -> (61.2, 0)
  line L5 (61.2, 0) -> (42.8, 0)
  line L6 (42.8, 0) -> (42.8, 6)
  line L7 (42.8, 6) -> (61.2, 6)
  line L8 (61.2, 6) -> (61.2, 0)
  line L9 (128, 0) -> (118.8, 0)
  line L10 (118.8, 0) -> (137.2, 0)
  line L11 (137.2, 0) -> (137.2, 6)
  line L12 (137.2, 6) -> (118.8, 6)
  line L13 (118.8, 6) -> (118.8, 0)
  point P0 (137.2, 0)
  point P1 (42.8, 0)
  dimension "d302" = 38
  dimension "d304" = 18.4
  dimension "d305" = 6
  dimension "d306" = 9.2
  constraints: 24 end point, 7 symmetric about line, 3 midpoint, 3 point on line, 2 parallel, 1 horizontal, 1 perpendicular, 1 vertical
  measures "d302" distance of L4.start L2.start
  measures "d304" distance of L7.start L7.end
  measures "d305" distance of L5.end L6.end
  measures "d306" distance of L4.end point (52, 0)
extrude "Extrusión19" cut sketch "Boceto23" against normal blind 12
sketch "Boceto24" plane through (-130, 0, -180) normal (-1, 0, 0) x (0, 0, 1)
  line L0 (0, 0) -> (180, 0) projected
  line L1 (90, 0) -> (90, 12)
  line L2 (177, 12) -> (3, 12) projected
  line L3 (61.2, 0) -> (42.8, 0)
  line L4 (42.8, 0) -> (42.8, 6)
  line L5 (42.8, 6) -> (61.2, 6)
  line L6 (61.2, 6) -> (61.2, 0)
  line L7 (118.8, 0) -> (137.2, 0)
  line L8 (137.2, 0) -> (137.2, 6)
  line L9 (137.2, 6) -> (118.8, 6)
  line L10 (118.8, 6) -> (118.8, 0)
  point P0 (52, 0)
  point P1 (128, 0)
  point P2 (137.2, 0)
  point P3 (42.8, 0)
  dimension "d311" = 38
  dimension "d312" = 9.2
  dimension "d313" = 18.4
  dimension "d314" = 6
  constraints: 18 end point, 5 symmetric about line, 3 midpoint, 2 parallel, 2 point on line, 1 horizontal, 1 perpendicular
  measures "d311" distance of point (90, 0) point (52, 0)
  measures "d312" distance of L3.start point (52, 0)
  measures "d313" distance of L4.end L5.end
  measures "d314" distance of L3.end L4.end
extrude "Extrusión20" cut sketch "Boceto24" against normal blind 12
